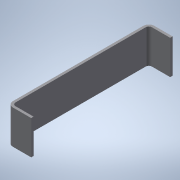
# Autodesk Inventor part: Fischer FME 7 Hood Profile Slice25mm
Saved by Autodesk Inventor 2022 (Build 260153000, 153)
## iProperties
Created: 2022-10-27
Part Number: Fischer FME 7 Hood Profile Slice25mm
Material: Generic
Document SubType Name: Modeling
Designer: baaij
Density: 1 g/cm^3
Appearance: Default
Author: baaij
Autodesk Inventor part; units mm, degrees
ref_plane "YZ Plane" through (0, 0, 0) normal (1, 0, 0) x (0, 1, 0)
ref_plane "XZ Plane" through (0, 0, 0) normal (0, 1, 0) x (-1, 0, 0)
ref_plane "XY Plane" through (0, 0, 0) normal (0, 0, 1) x (1, 0, 0)
sketch "Sketch1" plane through (0, 0, 0) normal (0, 0, 1) x (1, 0, 0)
  line L0 (-3.1, -51.95) -> (-16.6, -51.95)
  line L1 (-20.6, -47.95) -> (-20.6, 47.95)
  line L2 (-16.6, 51.95) -> (-3.1, 51.95)
  line L3 (-3.1, -51.95) -> (-20.6, 51.95) construction
  line L4 (-20.6, -51.95) -> (-3.1, 51.95) construction
  arc A0 (-16.6, 51.95) -> (-20.6, 47.95) centre (-16.6, 47.95) ccw
  arc A1 (-20.6, -47.95) -> (-16.6, -51.95) centre (-16.6, -47.95) ccw
  line L5 (-16.6, 50.15) -> (-3.1, 50.15)
  line L6 (-3.1, -50.15) -> (-16.6, -50.15)
  line L7 (-18.8, -47.95) -> (-18.8, 47.95)
  line L8 (-3.1, 51.95) -> (-3.1, 50.15)
  line L9 (-3.1, -50.15) -> (-3.1, -51.95)
  line L10 (-3.1, 51.95) -> (-3.1, -50.15) construction
  arc A2 (-16.6, 50.15) -> (-18.8, 47.95) centre (-16.6, 47.95) ccw
  arc A3 (-18.8, -47.95) -> (-16.6, -50.15) centre (-16.6, -47.95) ccw
  point P0 (0, 0)
  point P1 (-11.85, 0)
  dimension "d3" = 103.9
  dimension "d4" = 51.95
  dimension "d6" = 4
  dimension "d7" = 4
  dimension "d9" = 1.8
  dimension "d10" = 1.8
  dimension "d11" = 1.8
  dimension "d14" = 15.7
  dimension "d16" = 2.2
  dimension "d17" = 2.2
  dimension "d22" = 3.1
  constraints: 22 end point, 8 point on circle, 8 tangent, 4 centre point, 4 parallel, 4 point on line, 2 horizontal, 2 midpoint, 2 perpendicular, 1 vertical
  measures "d3" distance between parallel lines of L2 L0
  measures "d4" distance from line of point (0, 0) L2
  measures "d6" radius of A0
  measures "d7" radius of A1
  measures "d9" distance between parallel lines of L7 L1
  measures "d10" distance between parallel lines of L5 L2
  measures "d11" distance between parallel lines of L0 L6
  measures "d14" distance between parallel lines of L10 L7
  measures "d16" radius of A2
  measures "d17" radius of A3
  measures "d22" distance from line of point (0, 0) L10
extrude "Extrusion1" add sketch "Sketch1" along normal blind 25
body "Solid1"
